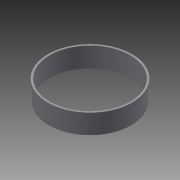
# Autodesk Inventor part: Top_Bevel_Base_Top
Saved by Autodesk Inventor 2015 (Build 190159000, 159)
## iProperties
Created: 2016-03-23
Part Number: Top_Bevel_Base_Top
Material: Generic
Document SubType Name: Modeling
Designer: david_000
Density: 1 g/cm^3
Appearance: Default
Author: david_000
Autodesk Inventor part; units mm, degrees
ref_plane "YZ Plane" through (0, 0, 0) normal (1, 0, 0) x (0, 1, 0)
ref_plane "XZ Plane" through (0, 0, 0) normal (0, 1, 0) x (-1, 0, 0)
ref_plane "XY Plane" through (0, 0, 0) normal (0, 0, 1) x (1, 0, 0)
sketch "Sketch1" plane through (0, 0, 0) normal (1, 0, 0) x (0, 1, 0)
  line L0 (0, 0) -> (0, -31.75)
  line L1 (0, -31.75) -> (3.175, -31.75)
  line L2 (3.175, -31.75) -> (3.175, -3.175)
  line L3 (114.3, -3.175) -> (114.3, 0)
  line L4 (114.3, 0) -> (0, 0)
  line L5 (72.0056, 146.05) -> (114.3, 146.05)
  line L6 (114.3, -3.175) -> (114.3, -6.35)
  line L7 (114.3, -6.35) -> (101.6, -6.35)
  line L8 (101.6, -6.35) -> (101.6, -3.175)
  line L9 (101.6, -3.175) -> (3.175, -3.175)
  line L10 (41.275, -3.175) -> (41.275, -1.5875)
  line L11 (41.275, -1.5875) -> (44.45, -1.5875)
  line L12 (44.45, -1.5875) -> (44.45, 0)
  dimension "d0" = 31.75
  dimension "d1" = 3.175
  dimension "d2" = 28.575
  dimension "d3" = 111.125
  dimension "d4" = 3.175
  dimension "d5" = 146.05
  dimension "d6" = 3.175
  dimension "d7" = 12.7
  dimension "d8" = 41.275
  dimension "d9" = 3.175
  constraints: 26 end point, 7 perpendicular, 3 vertical, 2 point on line, 1 horizontal
  measures "d0" distance of L0.start L1.start
  measures "d1" distance of L1.start L2.start
  measures "d2" distance of L2.start L2.end
  measures "d3" distance of L2.end L3.start
  measures "d4" distance of L3.start L4.start
  measures "d5" vertical distance of L0.start L5.start
  measures "d6" distance of L3.start L6.end
  measures "d7" distance of L6.end L7.end
  measures "d8" distance from line of L0 L10.start
  measures "d9" distance of L10.end L12.start
revolve "Revolution1" add sketch "Sketch1" angle 360 about axis through (0, 72.0056, 146.05) along (0, 1, 0) contours L4 L3 L6 L7 L8 L9 L10 L11 L12
body "Solid1"
